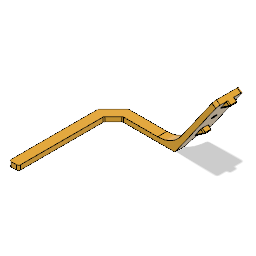
new_spool_limit v3 (Autodesk Fusion 360 design; units mm, degrees)
Autodesk Fusion 360 part; units mm, degrees
sketch "Sketch1" plane through (0, 0, 0) normal (1, 0, 0) x (0, 0, -1)
  line L0 (14, -30) -> (-14, -30)
  line L1 (-14, -30) -> (-14, 30)
  line L2 (-14, 30) -> (14, 30)
  line L3 (14, 30) -> (14, -30)
  line L4 (14, -30) -> (-14, 30) construction
  line L5 (-14, -30) -> (14, 30) construction
  line L6 (-114, 105) -> (-19.8579, 105)
  line L7 (-24, 95) -> (-114, 95)
  line L8 (-114, 95) -> (-114, 105)
  line L9 (-14, 85) -> (-14, 30)
  line L10 (-4, 89.1421) -> (-4, 30)
  line L11 (-24, 95) -> (-14, 85)
  line L12 (-19.8579, 105) -> (-4, 89.1421)
  line L13 (0, 30) -> (0, -30) construction
  circle A0 centre (0, 0) radius 2.7
  line L14 (-4.05, -17) -> (4.05, -17)
  line L15 (4.05, -17) -> (4.05, -30)
  line L16 (4.05, -30) -> (-4.05, -30)
  line L17 (-4.05, -30) -> (-4.05, -17)
  line L18 (-9.584, 30) -> (9.584, 30)
  line L19 (-4.05, 30) -> (4.05, 30)
  line L20 (4.05, 30) -> (4.05, 17)
  line L21 (4.05, 17) -> (-4.05, 17)
  line L22 (-4.05, 17) -> (-4.05, 30)
  circle A1 centre (14, 48) radius 18
  line L23 (-14, 48) -> (-4, 48)
  dimension "d1" = 28
  dimension "d2" = 60
  dimension "d4" = 10
  dimension "d5" = 10
  dimension "d6" = 10
  dimension "d7" = 65
  dimension "d8" = 10
  dimension "d9" = 45
  dimension "d10" = 100
  dimension "d11" = 5.4
  dimension "d19" = 8.1
  dimension "d20" = 13
  dimension "d22" = 8.1
  dimension "d23" = 13
  constraint horizontal L0
  constraint perpendicular L0 L1
  constraint parallel L0 L2
  constraint parallel L1 L3
  constraint coincident L4 A0.centre
  constraint coincident L5 A0.centre
  constraint coincident A0.centre origin
  constraint horizontal L6
  constraint horizontal L7
  constraint vertical L8
  constraint perpendicular L2 L9
  constraint coincident L2 L10.end
  constraint perpendicular L2 L10
  constraint parallel L11 L12
  constraint midpoint L2 L13.start
  constraint midpoint L0 L13.end
  constraint coincident L13 A0.centre
  constraint horizontal L14
  constraint vertical L15
  constraint horizontal L16
  constraint vertical L17
  constraint midpoint L13.end L16
  constraint horizontal L18
  constraint midpoint L13.start L18
  constraint horizontal L19
  constraint vertical L20
  constraint horizontal L21
  constraint vertical L22
  constraint midpoint L13.start L19
  constraint tangent L10 A1
  constraint tangent L2 A1
  constraint coincident L3 A1.centre
  constraint coincident L9 L23.start
  constraint coincident L10 L23.end
  constraint perpendicular L10 L23
  constraint coincident A1.centre L23
  measures "d1" distance of L0.start L0.end
  measures "d2" distance of L0.start L2.end
  measures "d4" distance of L6 L7
  measures "d5" distance of L9 L10
  measures "d6" distance of L11 L12
  measures "d7" distance of L2 L7
  measures "d8" distance of L7.start L9
  measures "d9" angle of L10 L12
  measures "d10" distance of L8 L9
  measures "d11" diameter of A0
  measures "d19" distance of L15.end L16.end
  measures "d20" distance of L14.start L16.end L0.start
  measures "d22" distance of L20.end L21.end
  measures "d23" distance of L19.start L21.end
  measures "d31" distance of L11
extrude "Extrude1" add sketch "Sketch1" along normal blind 5 contours L0 L1 L2 L3 L14 L15 L17 L18 L20 L21 L22 | L0 L14 L15 L16 L17 | L2 L10 L18 L19 A1 | L2 L9 L10 L18 L19 L23 | L2 L18 L19 L20 L21 L22
extrude "Extrude2" add sketch "Sketch1" against normal blind 5 contours L0 L14 L15 L16 L17 | L2 L18 L19 L20 L21 L22
ref_plane "WorkPlane1" through (0, 48, 9) normal (-0.573576, 0.819152, 0) x (0, 0, -1)
sketch "Sketch2" plane through (0, 48, 9) normal (-0.573576, 0.819152, 0) x (0, 0, -1)
  line L0 (5, 0) -> (-5, 0)
  line L1 (-5, 0) -> (-5, -55)
  line L2 (-5, -55) -> (-15, -65)
  line L3 (-15, -65) -> (-105, -65)
  line L4 (-105, -65) -> (-105, -75)
  line L5 (-105, -75) -> (-10.8579, -75)
  line L6 (-10.8579, -75) -> (5, -59.1421)
  line L7 (5, -59.1421) -> (5, 0)
  dimension "d31" = 10
  dimension "d34" = 10
  dimension "d35" = 65
  dimension "d36" = 135
  dimension "d37" = 10
  dimension "d38" = 10
  dimension "d39" = 100
  constraint coincident L0.end L1.start
  constraint perpendicular L1 L3
  constraint perpendicular L3 L4
  constraint perpendicular L1 L5
  constraint parallel L2 L6
  constraint coincident L0.start L7.end
  constraint parallel L1 L7
  constraint perpendicular L0 L1
  measures "d31" distance of L0.start L0.end
  measures "d34" distance of L1 L2.end
  measures "d35" distance of L0.end L3
  measures "d36" angle of L1 L2
  measures "d37" distance of L3.end L4.end
  measures "d38" distance of L2 L6
  measures "d39" distance of L1 L4
extrude "Extrude3" add sketch "Sketch2" against normal blind 5
fillet "Fillet4" radius 30 1 edges at (5, 45.3972, 9)
sketch "Sketch3" plane through (0, 0, 4.05) normal (0, 0, 1) x (1, 0, 0)
  line L0 (0, 17) -> (0, 30)
  line L1 (0, 30) -> (-5, 30)
  line L2 (-5, 30) -> (-5, 17)
  line L3 (-5, 17) -> (0, 17)
  line L4 (0, 30) -> (-5, 17)
  constraint coincident L0.end L1.start
  constraint coincident L2.end L3.start
extrude "Extrude4" cut sketch "Sketch3" against normal through all contours L1 L2 L4
sketch "Sketch4" plane through (0, 0, 4.05) normal (0, 0, 1) x (1, 0, 0)
  line L0 (0, -30) -> (0, -17)
  line L1 (0, -17) -> (-5, -17)
  line L2 (-5, -17) -> (-5, -30)
  line L3 (-5, -30) -> (0, -30)
  line L4 (0, -17) -> (-5, -30)
  constraint coincident L0.end L1.start
  constraint coincident L2.end L3.start
extrude "Extrude5" cut sketch "Sketch4" against normal through all contours L1 L2 L4
fillet "Fillet5" radius 3 3 edges at (2.5, 30, -14) (2.5, -30, -14) (2.5, -30, 14)
fillet "Fillet6" radius 2 6 edges at (62.8703, 88.9704, 114) (54.6788, 83.2346, 114) (54.6788, 83.2346, 24) (46.4873, 77.4988, 14) (49.8803, 79.8747, 4) (62.8703, 88.9704, 19.8579)
chamfer "Chamfer4" distance 1 angle 45 10 edges at (-2.5, -23.5, -4.05) (-2.5, -30, -4.05) (-2.5, -30, 4.05) (-2.5, -23.5, 4.05) (-5, -30, 0) (-5, 17, 0) (-2.5, 17, -4.05) (-2.5, 17, 4.05) (-2.5, 23.5, 4.05) (-2.5, 23.5, -4.05)
move_body "Move1" bodies 1 to x (-0.819152, 0.573576, 0) y (-0.573576, -0.819152, 0) z (0, 0, 1) at (0, 0, 0)
equation "d22 = d19"
